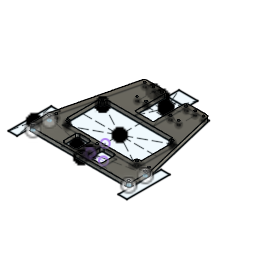
Base Plate v1 (Autodesk Fusion 360 design; units mm, degrees)
Autodesk Fusion 360 part; units mm, degrees
sketch "Sketch1" plane through (0, 0, 0) normal (0, 0, 1) x (1, 0, 0)
  line L0 (13, 77) -> (-13, 77)
  line L1 (-13, 77) -> (-13, 139)
  line L2 (-13, 139) -> (13, 139)
  line L3 (13, 139) -> (13, 77)
  line L4 (13, 77) -> (-13, 139) construction
  line L5 (-13, 77) -> (13, 139) construction
  line L6 (0, 1.75) -> (0, 22.5) construction
  line L7 (-13, 108) -> (-17, 108) construction
  line L8 (-17, 119) -> (-17, 97) construction
  circle A0 centre (-17, 119) radius 1.65
  circle A1 centre (-17, 97) radius 1.65
  circle A2 centre (17, 97) radius 1.65
  circle A3 centre (17, 119) radius 1.65
  line L9 (71, -15) -> (-71, -15)
  line L10 (-71, -15) -> (-71, 15)
  line L11 (-71, 15) -> (71, 15) construction
  line L12 (71, 15) -> (71, -15)
  line L13 (71, -15) -> (-71, 15) construction
  line L14 (-71, -15) -> (71, 15) construction
  circle A4 centre (-67.158, 11.4917) radius 1.65
  line L15 (0, 15) -> (0, -15) construction
  circle A5 centre (0, -11) radius 1.7
  line L16 (20, 0) -> (2.5, 0) construction
  circle A6 centre (0, 11) radius 1.7
  line L17 (-7, 15) -> (-7, -15) construction
  line L18 (-7, 11) -> (-27, 11)
  line L19 (-27, 11) -> (-27, -11)
  line L20 (-27, -11) -> (-7, -11)
  line L21 (-7, -11) -> (-7, 11)
  line L22 (-7, 11) -> (-27, -11) construction
  line L23 (-27, 11) -> (-7, -11) construction
  line L24 (27, 11) -> (27, -11)
  line L25 (27, -11) -> (7, -11)
  line L26 (7, -11) -> (7, 11)
  line L27 (7, 11) -> (27, 11)
  circle A7 centre (-67.158, -11.4917) radius 1.65
  circle A8 centre (67.158, 11.4917) radius 1.65
  circle A9 centre (67.158, -11.4917) radius 1.65
  line L28 (-83, 30) -> (-71, 30)
  line L29 (-71, 30) -> (-71, -30)
  line L30 (-71, -30) -> (-83, -30)
  line L31 (-83, -30) -> (-83, 30)
  line L32 (-83, 30) -> (-71, -30) construction
  line L33 (-71, 30) -> (-83, -30) construction
  line L34 (83, 30) -> (71, 30)
  line L35 (71, 30) -> (71, -30)
  line L36 (83, -30) -> (83, 30)
  line L37 (71, -30) -> (83, -30)
  line L38 (-45, 123) -> (45, 123)
  line L39 (0, 123) -> (0, 108) construction
  line L40 (-45, 123) -> (-71, 15)
  line L41 (45, 123) -> (71, 15)
  line L42 (0, 77) -> (0, 15) construction
  line L43 (-52, 71) -> (52, 71)
  line L44 (52, 71) -> (52, 15)
  line L45 (52, 15) -> (-52, 15)
  line L46 (-52, 15) -> (-52, 71)
  line L47 (-52, 71) -> (52, 15) construction
  line L48 (52, 71) -> (-52, 15) construction
  circle A10 centre (-49, 68) radius 1.5
  circle A11 centre (49, 68) radius 1.5
  line L49 (-52, 43) -> (52, 43) construction
  circle A12 centre (49, 18) radius 1.5
  circle A13 centre (-49, 18) radius 1.5
  line L50 (-52, 71) -> (-46, 71) construction
  line L51 (-46, 71) -> (-46, 65)
  line L52 (-46, 65) -> (-52, 65)
  line L53 (-52, 65) -> (-52, 71) construction
  line L54 (-52, 71) -> (-46, 65) construction
  line L55 (-46, 71) -> (-52, 65) construction
  line L56 (46, 65) -> (52, 65)
  line L57 (46, 71) -> (46, 65)
  line L58 (46, 21) -> (52, 21)
  line L59 (46, 15) -> (46, 21)
  line L60 (-46, 15) -> (-46, 21)
  line L61 (-46, 21) -> (-52, 21)
  circle A14 centre (-41, 119) radius 1.5
  circle A15 centre (41, 119) radius 1.5
  circle A16 centre (-65, 19) radius 1.5
  circle A17 centre (65, 19) radius 1.5
  line L62 (-29, 119.5) -> (29, 119.5) construction
  line L63 (29, 119.5) -> (29, 96.5) construction
  line L64 (29, 96.5) -> (-29, 96.5) construction
  line L65 (-29, 96.5) -> (-29, 119.5) construction
  line L66 (-29, 119.5) -> (29, 96.5) construction
  line L67 (29, 119.5) -> (-29, 96.5) construction
  circle A18 centre (-29, 119.5) radius 1.4
  circle A19 centre (29, 119.5) radius 1.4
  circle A20 centre (29, 96.5) radius 1.4
  circle A21 centre (-29, 96.5) radius 1.4
  point P0 (0, 108)
  point P1 (-17, 0)
  point P2 (-77, 0)
  point P3 (0, 43)
  point P4 (-49, 68)
  point P5 (0, 108)
  dimension "d1" = 26
  dimension "d2" = 62
  dimension "d3" = 4
  dimension "d4" = 3.3
  dimension "d5" = 142
  dimension "d6" = 30
  dimension "d8" = 3.3
  dimension "d9" = 3.4
  dimension "d10" = 4
  dimension "d11" = 7
  dimension "d12" = 20
  dimension "d13" = 22
  dimension "d14" = 12
  dimension "d15" = 60
  dimension "d16" = 62
  dimension "d17" = 4
  dimension "d18" = 22
  dimension "d19" = 28
  dimension "d20" = 104
  dimension "d21" = 56
  dimension "d22" = 3
  dimension "d23" = 3
  dimension "d24" = 3
  dimension "d33" = 3
  dimension "d34" = 4
  dimension "d35" = 24
  dimension "d36" = 3
  dimension "d37" = 4
  dimension "d38" = 16
  dimension "d39" = 58
  dimension "d40" = 23
  dimension "d41" = 2.8
  constraint horizontal L0
  constraint perpendicular L0 L1
  constraint parallel L0 L2
  constraint parallel L1 L3
  constraint coincident L4 P0
  constraint coincident L5 P0
  constraint coincident P0 L6
  constraint perpendicular L1 L7
  constraint perpendicular L7 L8
  constraint midpoint L7.end L8
  constraint midpoint L1 L7.start
  constraint coincident L8.start A0.centre
  constraint symmetric L7 A0 A1
  constraint symmetric L6 A0 A3
  constraint symmetric L6 A1 A2
  constraint horizontal L9
  constraint perpendicular L9 L10
  constraint parallel L9 L11
  constraint parallel L10 L12
  constraint coincident L13 origin
  constraint coincident L14 origin
  constraint midpoint L11 L15.start
  constraint midpoint L9 L15.end
  constraint coincident L15 A5.centre
  constraint symmetric A5 L16 A6
  constraint coincident L11 L17.start
  constraint coincident L9 L17.end
  constraint perpendicular L9 L17
  constraint horizontal L18
  constraint perpendicular L18 L19
  constraint parallel L18 L20
  constraint parallel L19 L21
  constraint coincident L22 P1
  constraint coincident L23 P1
  constraint midpoint L17 L21
  constraint symmetric L15 L18.start L26.end
  constraint symmetric L15 L18.end L24.start
  constraint symmetric L15 L19.end L24.end
  constraint symmetric L15 L20.end L25.end
  constraint symmetric A4 L16 A7
  constraint symmetric L6 A4 A8
  constraint symmetric L6 A7 A9
  constraint horizontal L28
  constraint perpendicular L28 L29
  constraint parallel L28 L30
  constraint parallel L29 L31
  constraint coincident L32 P2
  constraint coincident L33 P2
  constraint midpoint L10 L29
  constraint symmetric L6 L28.start L34.start
  constraint symmetric L6 L28.end L34.end
  constraint symmetric L6 L29.end L35.end
  constraint symmetric L6 L30.end L36.start
  constraint perpendicular L1 L38
  constraint midpoint L38 L39.start
  constraint coincident P0 L39.end
  constraint vertical L39
  constraint midpoint L0 L42.start
  constraint horizontal L43
  constraint perpendicular L43 L44
  constraint parallel L43 L45
  constraint parallel L44 L46
  constraint coincident L47 P3
  constraint coincident L48 P3
  constraint symmetric L42 A10 A11
  constraint midpoint L46 L49.start
  constraint midpoint L44 L49.end
  constraint symmetric A10 L49 A13
  constraint symmetric A11 L49 A12
  constraint horizontal L50
  constraint perpendicular L50 L51
  constraint parallel L50 L52
  constraint parallel L51 L53
  constraint coincident L54 P4
  constraint coincident L55 P4
  constraint coincident P4 A10.centre
  constraint symmetric L42 L50.end L57.start
  constraint symmetric L42 L51.end L56.start
  constraint symmetric L42 L52.end L56.end
  constraint symmetric L49 L50.end L60.start
  constraint symmetric L49 L51.end L60.end
  constraint symmetric L49 L52.end L61.end
  constraint symmetric L49 L56.start L58.start
  constraint symmetric L49 L56.end L58.end
  constraint symmetric L49 L57.start L59.start
  constraint coincident L42 P3
  constraint midpoint L11 L45
  constraint symmetric L39 A14 A15
  constraint symmetric L42 A16 A17
  constraint horizontal L62
  constraint perpendicular L62 L63
  constraint parallel L62 L64
  constraint parallel L63 L65
  constraint coincident L66 P5
  constraint coincident L67 P5
  constraint coincident L62.start L65.end
  constraint symmetric L39 A18 A19
  constraint symmetric L7 A18 A21
  constraint symmetric L7 A19 A20
  measures "d1" distance of L1.end L2.end
  measures "d2" distance of L0.end L1.end
  measures "d3" distance of L7.start L7.end
  measures "d4" diameter of A0
  measures "d5" distance of L10.end L11.end
  measures "d6" distance of L9.end L10.end
  measures "d8" diameter of A4
  measures "d9" diameter of A5
  measures "d10" distance of L9 A5.centre
  measures "d11" distance of origin L17
  measures "d12" distance of L19.end L20.end
  measures "d13" distance of L18.end L19.end
  measures "d14" distance of L29.end L30.end
  measures "d15" distance of L28.end L29.end
  measures "d16" distance of L0 L11
  measures "d17" distance of L8.start L38
  measures "d18" distance of L8.start L8.end
  measures "d19" horizontal distance of L8.start L38.start
  measures "d20" distance of L43.start L43.end
  measures "d21" distance of L43.start L45.end
  measures "d22" diameter of A10
  measures "d23" distance of L43 P4
  measures "d24" distance of L46 P4
  measures "d33" diameter of A14
  measures "d34" distance of L38 A14.centre
  measures "d35" distance of L8.start A14.centre
  measures "d36" diameter of A16
  measures "d37" distance of L11 A16.centre
  measures "d38" horizontal distance of A13.centre A16.centre
  measures "d39" distance of L63.end L64.end
  measures "d40" distance of L62.end L63.end
  measures "d41" diameter of A18
extrude "Extrude1" add sketch "Sketch1" along normal blind 5.6 contours L0 L1 L3 L9 L10 L12 L29 L35 L38 L40 L41 | L43 L46 L51 L52 | L43 L44 L56 L57 | L45 L46 L60 L61 | L44 L45 L58 L59
fillet "Fillet1" radius 3 12 edges at (-46, 65, 2.8) (46, 65, 2.8) (46, 21, 2.8) (-46, 21, 2.8) (27, -11, 2.8) (7, -11, 2.8) (7, 11, 2.8) (27, 11, 2.8) (-7, 11, 2.8) (-27, 11, 2.8) (-27, -11, 2.8) (-7, -11, 2.8)
fillet "Fillet2" radius 1 2 edges at (13, 77, 2.8) (-13, 77, 2.8)
fillet "Fillet3" radius 4 8 edges at (45, 123, 2.8) (-45, 123, 2.8) (71, 15, 2.8) (-71, 15, 2.8) (71, -15, 2.8) (-71, -15, 2.8) (-13, 123, 2.8) (13, 123, 2.8)
equation "d5 = ( ( 70 * 2 ) * 1 ) * 1 mm + 2 mm"
equation "d20 = ( 13 * 8 ) * 1 mm"
